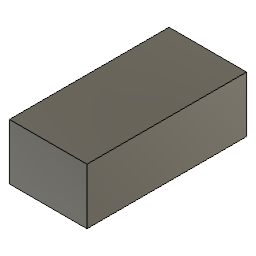
SENIOR_FINAL_CASE (Autodesk Fusion 360 design; units mm, degrees)
part number: 2026-04-21-16-02-39-932
Autodesk Fusion 360 part; units mm, degrees
note: some values were not read from the file. Set by a fixed rule: which face or edge a step refers to.
sketch "Sketch1" plane through (0, 0, 0) normal (0, 0, 1) x (1, 0, 0)
  line L0 (0, 0) -> (110, 0)
  line L1 (110, 0) -> (110, 220)
  line L2 (110, 220) -> (0, 220)
  line L3 (0, 220) -> (0, 0)
  dimension "d1" = 110
  dimension "d2" = 220
  constraint horizontal L0
  constraint vertical L1
  constraint horizontal L2
  constraint vertical L3
  constraint coincident L0.start L3.end
  measures "d1" distance of L0.start L0.end
  measures "d2" distance of L0.start L2.end
extrude "Extrude1" add sketch "Sketch1" along normal blind 145 makes body 1
shell "Shell1" thickness 3 removed faces 1 at (36.6667, 146.6667, 145) on bodies 1
move_face "OffsetFaces1" offset -2.5 1 faces at (37.6667, 74.3333, 3) on bodies 1
sketch "Sketch2" plane through (0, 0, 0.5) normal (0, 0, 1) x (-1, 0, 0)
  line L0 (-3, -217) -> (-3, -3)
  line L1 (-3, -3) -> (-107, -3)
  line L2 (-107, -3) -> (-107, -217)
  line L3 (-107, -217) -> (-3, -217)
  line L4 (-3, -3) -> (-107, -3)
  line L5 (-107, -3) -> (-107, -217)
  line L6 (-107, -217) -> (-3, -217)
  line L7 (-3, -217) -> (-3, -3)
  constraint horizontal L4
  constraint vertical L5
  constraint horizontal L6
  constraint vertical L7
  constraint coincident L2.end L3.start
  constraint coincident L0.end L1.start
extrude "Extrude2" add sketch "Sketch2" along normal blind 75 separate body makes body 2
sketch "Sketch3" plane through (0, 0, 75.5) normal (0, 0, 1) x (-1, 0, 0)
  line L0 (-3, -217) -> (-3, -3)
  line L1 (-3, -3) -> (-107, -3)
  line L2 (-107, -3) -> (-107, -217)
  line L3 (-107, -217) -> (-3, -217)
  line L4 (-3, -3) -> (-11.5, -3)
  line L5 (-11.5, -3) -> (-11.5, -14)
  line L6 (-107, -3) -> (-98.5, -3)
  line L7 (-98.5, -3) -> (-98.5, -14)
  line L8 (-3, -217) -> (-11.5, -217)
  line L9 (-11.5, -217) -> (-11.5, -206)
  line L10 (-107, -217) -> (-98.5, -217)
  line L11 (-98.5, -217) -> (-98.5, -206)
  line L12 (-11.5, -14) -> (-98.5, -14)
  line L13 (-98.5, -14) -> (-98.5, -206)
  line L14 (-98.5, -206) -> (-11.5, -206)
  line L15 (-11.5, -206) -> (-11.5, -14)
  dimension "d9" = 8.5
  dimension "d10" = 11
  dimension "d11" = 8.5
  dimension "d12" = 11
  dimension "d13" = 8.5
  dimension "d14" = 11
  dimension "d15" = 8.5
  dimension "d16" = 11
  constraint coincident L0.end L1.start
  constraint perpendicular L0 L4
  constraint perpendicular L1 L5
  constraint coincident L1.end L2.start
  constraint perpendicular L2 L6
  constraint perpendicular L6 L7
  constraint coincident L0.start L3.end
  constraint perpendicular L0 L8
  constraint perpendicular L3 L9
  constraint coincident L2.end L3.start
  constraint perpendicular L2 L10
  constraint perpendicular L3 L11
  constraint horizontal L12
  constraint vertical L13
  constraint horizontal L14
  constraint vertical L15
  measures "d9" distance of L0.end L4.end
  measures "d10" distance of L4.end L5.end
  measures "d11" distance of L1.end L6.end
  measures "d12" distance of L6.end L7.end
  measures "d13" distance of L0.start L8.end
  measures "d14" distance of L8.end L9.end
  measures "d15" distance of L2.end L10.end
  measures "d16" distance of L10.end L11.end
extrude "Extrude3" add sketch "Sketch3" along normal blind 2 separate body contours L12 L13 L14 L15 makes body 3
move_face "OffsetFaces2" offset -2.5 1 faces at (36.6667, 0, 48.3333) on bodies 1
move_face "OffsetFaces3" offset -2.5 1 faces at (37.6667, 217, 96.8333) on bodies 1
hidden bodies 1 3
named bodies: "CASE", "REF_BATT", "REF_PCB"
